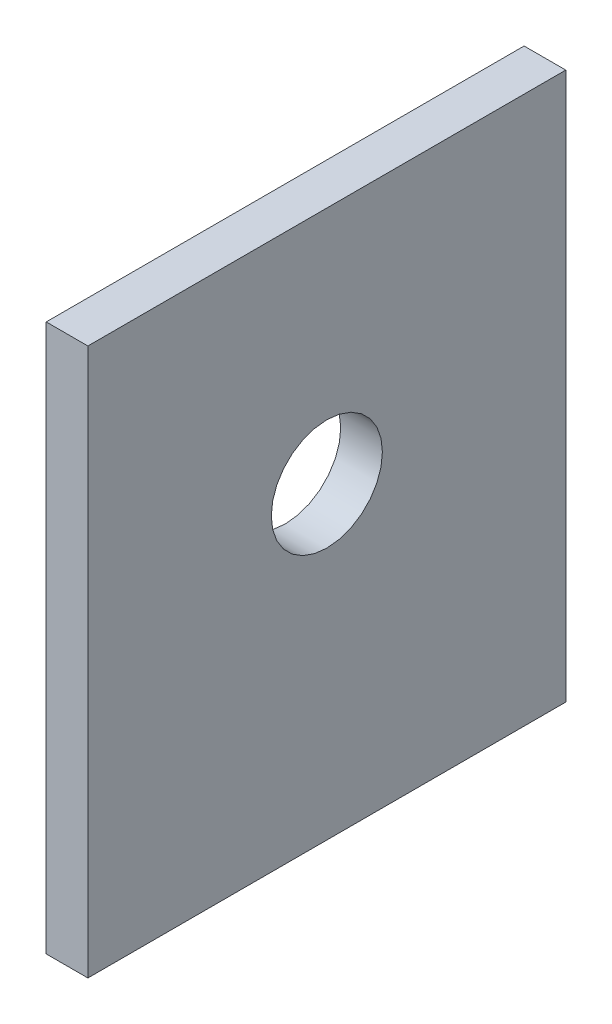
# Autodesk Inventor part: cord roller
Saved by Autodesk Inventor 2023 (Build 270158000, 158)
## iProperties
Created: 2023-02-17
Part Number: cord roller
Material: Generic
Document SubType Name: Modeling
Designer: shrey
Density: 1 g/cm^3
Appearance: Default
Author: shrey
Autodesk Inventor part; units mm, degrees
ref_plane "YZ Plane" through (0, 0, 0) normal (1, 0, 0) x (0, 1, 0)
ref_plane "XZ Plane" through (0, 0, 0) normal (0, 1, 0) x (-1, 0, 0)
ref_plane "XY Plane" through (0, 0, 0) normal (0, 0, 1) x (1, 0, 0)
ref_plane "Work Plane1" through (0, 0, -290) normal (1, 0, 0) x (0, 1, 0)
sketch "Sketch1" plane through (0, 0, -290) normal (1, 0, 0) x (0, 1, 0)
  circle A0 centre (-627.5, 172.5) radius 11 construction
  circle A1 centre (-627.5, 172.5) radius 4 construction
  line L0 (-655, 150) -> (-605, 150)
  line L1 (-605, 150) -> (-605, 195)
  line L2 (-605, 195) -> (-655, 195)
  line L3 (-655, 195) -> (-655, 150)
  circle A2 centre (-627.5, 172.5) radius 16 construction
  line L4 (0, 0) -> (-700, 0) projected
  line L5 (-700, -55) -> (-700, 580) projected
  circle A3 centre (-627.5, 172.5) radius 4
  line L6 (-649.7, 155.3) -> (-610.3, 155.3)
  line L7 (-610.3, 155.3) -> (-610.3, 189.7)
  line L8 (-610.3, 189.7) -> (-649.7, 189.7)
  line L9 (-649.7, 189.7) -> (-649.7, 155.3)
  point P0 (0, 290)
  dimension "d0" = 22
  dimension "d1" = 8
  dimension "d2" = 45
  dimension "d3" = 50
  dimension "d4" = 5
  dimension "d7" = 22.5
  dimension "d8" = 22.5
  dimension "d10" = 5.3
  dimension "d13" = 150
  dimension "d14" = 95
  constraints: 16 end point, 4 centre point, 4 parallel, 2 coincident, 2 perpendicular, 1 concentric, 1 horizontal, 3 other
  measures "d0" diameter of A0
  measures "d1" diameter of A1
  measures "d2" distance of L0.end L1.end
  measures "d3" distance of L0.start L0.end
  measures "d4" radial gap between concentric circles of A0 A2
  measures "d7" distance from line of L1 A0.centre
  measures "d8" distance from line of L0 A0.centre
  measures "d10" distance between parallel lines of L3 L9
  measures "d13" distance between parallel lines of L4 L0
  measures "d14" distance between parallel lines of L5 L1
extrude "Extrusion1" add sketch "Sketch1" along normal blind 3 contours L9 L8 L7 L6
body "Solid1"
